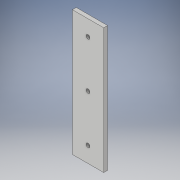
# Autodesk Inventor part: 1x4x.125bar
Saved by Autodesk Inventor 2018 (Build 220112000, 112)
## iProperties
Created: 2018-08-04
Part Number: 1x4x.125bar
Material: Generic
Document SubType Name: Modeling
Designer: Cole Tucker
Density: 1 g/cm^3
Appearance: Default
Author: Cole Tucker
Autodesk Inventor part; units mm, degrees
ref_plane "YZ Plane" through (0, 0, 0) normal (1, 0, 0) x (0, 1, 0)
ref_plane "XZ Plane" through (0, 0, 0) normal (0, 1, 0) x (-1, 0, 0)
ref_plane "XY Plane" through (0, 0, 0) normal (0, 0, 1) x (1, 0, 0)
sketch "Sketch1" plane through (0, 0, 0) normal (0, 0, 1) x (1, 0, 0)
  line L0 (0, 0) -> (25.4, 0)
  line L1 (25.4, 0) -> (25.4, 101.6)
  line L2 (25.4, 101.6) -> (0, 101.6)
  line L3 (0, 101.6) -> (0, 0)
  dimension "d0" = 25.4
  dimension "d1" = 101.6
  constraints: 8 end point, 2 parallel, 1 horizontal, 1 perpendicular
  measures "d0" distance of L2.end L1.end
  measures "d1" distance of L1.end L0.end
extrude "Extrusion1" add sketch "Sketch1" along normal blind 3.175
sketch "Sketch2" plane through (0, 0, 3.175) normal (0, 0, 1) x (1, 0, 0)
  line L0 (25.4, 101.6) -> (0, 101.6) projected
  line L1 (12.7, 101.6) -> (12.7, 88.9)
  line L2 (12.7, 50.8) -> (12.7, 12.7)
  line L3 (12.7, 88.9) -> (12.7, 50.8)
  point P0 (0, 0)
  dimension "d4" = 12.7
  dimension "d7" = 38.1
  dimension "d8" = 38.1
  constraints: 6 end point, 3 coincident, 2 vertical, 1 midpoint
  measures "d4" distance of L1.start L1.end
  measures "d7" distance of L2.start L2.end
  measures "d8" distance of L3.start L3.end
hole "Hole1" at (12.7, 88.9, 3.175) at (12.7, 50.8, 3.175) at (12.7, 12.7, 3.175) direction (0, 0, -1) diameter 3.175 depth 25.4 tip angle 118
body "Solid1"
